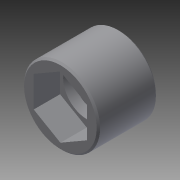
# Autodesk Inventor part: D-117199-bif
Saved by Autodesk Inventor 2014 SP2 (Build 180246200, 246)
## iProperties
Created: 2020-02-04
Part Number: D-117199-bif
Material: Generic
Catalog Web Link: www.cadenas.de
Description: BIF Nut-Bimba FLAT-1
Vendor: BIMBA
Document SubType Name: Modeling
Designer: psadmin
Manufacturer: BIMBA
Mass: 0.0677468 g
Surface Area: 1.57525 cm^2
Volume: 0.0677468 cm^3
Density: 1 g/cm^3
Appearance: PSOLRGB-192-192-192
Category: PARTsolutions
Company: BIMBA
Title: D-117199-bif
Author: Cadenas PARTsolutions
Comments: Bimba FLAT-1
PSOL_IDENT_0: {$CADENAS_DATA\23d-libs\bimba\bimba_brand\bimba_imperial\bimba_full_line\flat_cylinders\fo1\bif_nut.
PSOL_IDENT_1: prj},166 {VTYP=3D},{NB=D-117199-bif},{LINA=D-117199-bif},{NN=BIF Nut},{DATE=22.01.2020 09:06:06},{GE
PSOL_IDENT_2: OMDATE=09.03.2017 10:13:28},{VERSION=},{LINEID=100},{WBVAR=},{WBNUMERIC=}  {NB=D-117199-bif},{LINA=D
PSOL_IDENT_3: -117199-bif},{KT=DUMMY},{PN=D-117199},{NDM=0.138},{H=0.222},{HL=0.173},{HW=0.156},{HWL=0.077},{CH=0.
PSOL_IDENT_4: 005}
NN: BIF Nut
NT: Bimba FLAT-1
NB: D-117199-bif
NBSYN: $PN.-bif
LINA: D-117199-bif
PN: D-117199
NDM: 0.138
H: 0.222
HL: 0.173
HW: 0.156
HWL: 0.077
CH: 0.005
SUPPLIER: BIMBA
ARTICLENO: D-117199-bif
BOMINFO: D-117199-bif
CREATOR: CADENAS GmbH
Autodesk Inventor part; units mm, degrees
ref_plane "YZ Plane" through (0, 0, 0) normal (1, 0, 0) x (0, 1, 0)
ref_plane "XZ Plane" through (0, 0, 0) normal (0, 1, 0) x (-1, 0, 0)
ref_plane "XY Plane" through (0, 0, 0) normal (0, 0, 1) x (1, 0, 0)
sketch "Sketch_1" plane through (0, 0, 0) normal (1, 0, 0) x (0, 1, 0)
  line L0 (0, -4.3942) -> (0, 0)
  line L1 (1.7526, 0) -> (1.7526, -1.9558)
  line L2 (1.7526, -1.9558) -> (1.3233, -2.3851)
  line L3 (1.3233, -2.3851) -> (1.3233, -3.9649)
  line L4 (1.3233, -3.9649) -> (1.7526, -4.3942)
  line L5 (1.7526, -4.3942) -> (2.6924, -4.3942)
  line L6 (2.6924, -4.3942) -> (2.8194, -4.2672)
  line L7 (2.8194, -4.2672) -> (2.8194, -0.127)
  line L8 (2.8194, -0.127) -> (2.6924, 0)
  line L9 (2.6924, 0) -> (1.7526, 0)
  constraints: 20 end point
revolve "Revolution1" add sketch "Sketch_1" angle 360 about axis through (0, 0, -4.3942) along (0, 0, -1)
thread "Thread1" size "6-32 UNC" class "2B" standard "ANSI Unified Screw Threads" full length
sketch "Sketch_3" plane through (0, 0, 0) normal (0, 0, 1) x (1, 0, 0)
  line L0 (-1.9812, -1.1438) -> (0, -2.2877)
  line L1 (0, -2.2877) -> (1.9812, -1.1438)
  line L2 (1.9812, -1.1438) -> (1.9812, 1.1438)
  line L3 (1.9812, 1.1438) -> (0, 2.2877)
  line L4 (0, 2.2877) -> (-1.9812, 1.1438)
  line L5 (-1.9812, 1.1438) -> (-1.9812, -1.1438)
  constraints: 12 end point
extrude "Extrusion1" cut sketch "Sketch_3" against normal blind 1.9558
ref_plane "screw_XY" through (0, 0, -4.3942) normal (0, 0, 1) x (1, 0, 0)
ref_plane "screw_YZ" through (0, 0, -4.3942) normal (1, 0, 0) x (0, 1, 0)
ref_plane "screw_ZX" through (0, 0, -4.3942) normal (0, 1, 0) x (0, 0, 1)
body "Solid1"
